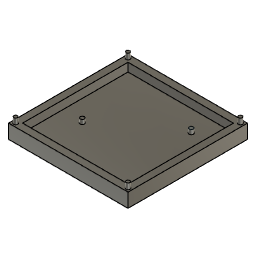
Untitled v0 (Autodesk Fusion 360 design; units mm, degrees)
Autodesk Fusion 360 part; units mm, degrees
note: some values were not read from the file. Set by a fixed rule: which sketch regions a step uses.
sketch "Sketch1" plane through (0, 0, 0) normal (0, 0, 1) x (1, 0, 0)
  line L0 (0, 0) -> (0, 75)
  line L1 (0, 75) -> (75, 75)
  line L2 (75, 75) -> (75, 0)
  line L3 (75, 0) -> (0, 0)
  line L4 (-5, -5) -> (-5, 80)
  line L5 (-5, 80) -> (80, 80)
  line L6 (80, 80) -> (80, -5)
  line L7 (80, -5) -> (-5, -5)
  dimension "d1" = 75
  dimension "d2" = 75
  dimension "d3" = 75
  dimension "d4" = 75
  dimension "d5" = 85
  dimension "d6" = 85
  dimension "d7" = 85
  dimension "d8" = 85
  constraint coincident L0.start L3.end
  constraint vertical L0
  constraint perpendicular L0 L1
  constraint perpendicular L1 L2
  constraint perpendicular L0 L3
  constraint parallel L0 L4
  constraint perpendicular L4 L5
  constraint perpendicular L5 L6
  constraint perpendicular L4 L7
  measures "d1" distance of L0.start L0.end
  measures "d2" distance of L0.end L1.end
  measures "d3" distance of L1.end L2.end
  measures "d4" distance of L2.end L0.start
  measures "d5" distance of L4.start L4.end
  measures "d6" distance of L4.end L5.end
  measures "d7" distance of L5.end L6.end
  measures "d8" distance of L6.end L4.start
extrude "Extrude1" add sketch "Sketch1" along normal blind 10
sketch "Sketch2" plane through (0, 0, 0) normal (0, 1, 0) x (1, 0, 0)
sketch "Sketch3" plane through (0, 0, 0) normal (0, 0, 1) x (1, 0, 0)
  line L0 (0, 0) -> (75, 0)
  line L1 (75, 0) -> (75, 75)
  line L2 (75, 75) -> (0, 75)
  line L3 (0, 75) -> (0, 0)
  constraint horizontal L0
  constraint vertical L1
  constraint horizontal L2
  constraint vertical L3
  constraint coincident L0.start L3.end
extrude "Extrude2" add sketch "Sketch3" along normal blind 4
sketch "Sketch4" plane through (0, 0, 4) normal (0, 0, 1) x (-1, 0, 0)
  line L0 (0, -75) -> (0, 0)
  line L1 (0, 0) -> (-75, 0)
  line L2 (-75, 0) -> (-75, -75)
  line L3 (-75, -75) -> (0, -75)
  line L4 (0, 0) -> (-75, -75)
  line L5 (-75, 0) -> (0, -75)
  line L6 (-37.5, -37.5) -> (-37.5, -65)
  line L7 (-37.5, -37.5) -> (-65, -37.5)
  line L8 (-65, -37.5) -> (-65, -10)
  line L9 (-37.5, -65) -> (-10, -65)
  line L10 (-10, -65) -> (-65, -65)
  line L11 (-65, -65) -> (-65, -10)
  line L12 (-65, -10) -> (-10, -10)
  line L13 (-10, -10) -> (-10, -65)
  line L14 (-65, -65) -> (-60, -65)
  line L15 (-60, -65) -> (-60, -60)
  circle A0 centre (-60, -60) radius 1.625
  line L16 (-10, -10) -> (-10, -27.5)
  line L17 (-10, -27.5) -> (-15, -27.5)
  circle A1 centre (-15, -27.5) radius 1.625
  dimension "d13" = 27.5
  dimension "d14" = 27.5
  dimension "d15" = 27.5
  dimension "d16" = 27.5
  dimension "d17" = 5
  dimension "d18" = 5
  dimension "d19" = 3.25
  dimension "d20" = 17.5
  dimension "d21" = 5
  dimension "d22" = 3.25
  constraint coincident L0.end L1.start
  constraint coincident L2.end L3.start
  constraint coincident L1.end L2.start
  constraint coincident L0.start L3.end
  constraint midpoint L4 L6.start
  constraint vertical L6
  constraint perpendicular L6 L7
  constraint perpendicular L7 L8
  constraint perpendicular L6 L9
  constraint horizontal L10
  constraint vertical L11
  constraint horizontal L12
  constraint vertical L13
  constraint perpendicular L11 L14
  constraint perpendicular L10 L15
  constraint coincident L15.end A0.centre
  constraint perpendicular L12 L16
  constraint perpendicular L13 L17
  constraint coincident L17.end A1.centre
  measures "d13" distance of L6.start L6.end
  measures "d14" distance of L6.start L7.end
  measures "d15" distance of L7.end L8.end
  measures "d16" distance of L6.end L9.end
  measures "d17" distance of L10.end L14.end
  measures "d18" distance of L14.end L15.end
  measures "d19" diameter of A0
  measures "d20" distance of L12.end L16.end
  measures "d21" distance of L16.end L17.end
  measures "d22" diameter of A1
extrude "Extrude3" add sketch "Sketch4" along normal blind 3 draft -4 contours L4 A0 | L4 L15 A0 | L4 L15 A0 | A1
sketch "Sketch5" plane through (0, 0, 10) normal (0, 0, 1) x (-1, 0, 0)
  line L0 (-75, -75) -> (-75, 0)
  line L1 (-75, 0) -> (0, 0)
  line L2 (0, 0) -> (0, -75)
  line L3 (0, -75) -> (-75, -75)
  line L4 (-80, 5) -> (-80, -80)
  line L5 (-80, -80) -> (5, -80)
  line L6 (5, -80) -> (5, 5)
  line L7 (5, 5) -> (-80, 5)
  line L8 (5, 5) -> (0, 0)
  line L9 (5, 0) -> (0, 5)
  circle A0 centre (2.5, 2.5) radius 1.5
  line L10 (-75, -75) -> (-80, -80)
  line L11 (-80, -75) -> (-75, -80)
  circle A1 centre (-77.5, -77.5) radius 1.5
  line L12 (0, -75) -> (5, -80)
  line L13 (5, -75) -> (0, -80)
  circle A2 centre (2.5, -77.5) radius 1.5
  line L14 (-80, 5) -> (-75, 0)
  line L15 (-75, 5) -> (-80, 0)
  circle A3 centre (-77.5, 2.5) radius 1.5
  dimension "d25" = 3
  dimension "d26" = 3
  dimension "d27" = 3
  dimension "d28" = 3
  constraint coincident L6.end L7.start
  constraint coincident L1.end L2.start
  constraint coincident L6 L9.start
  constraint coincident L7 L9.end
  constraint perpendicular L8 L9
  constraint midpoint L8 A0.centre
  constraint coincident L0.start L3.end
  constraint coincident L4.end L5.start
  constraint coincident L4 L11.start
  constraint coincident L5 L11.end
  constraint perpendicular L10 L11
  constraint midpoint L11 A1.centre
  constraint coincident L2.end L3.start
  constraint coincident L5.end L6.start
  constraint coincident L6 L13.start
  constraint coincident L5 L13.end
  constraint perpendicular L12 L13
  constraint midpoint L12 A2.centre
  constraint coincident L4.start L7.end
  constraint coincident L0.end L1.start
  constraint coincident L7 L15.start
  constraint coincident L4 L15.end
  constraint perpendicular L14 L15
  constraint midpoint L14 A3.centre
  measures "d25" diameter of A0
  measures "d26" diameter of A1
  measures "d27" diameter of A2
  measures "d28" diameter of A3
extrude "Extrude4" add sketch "Sketch5" along normal blind 4 draft -3 contours L10 L11 A1 | L10 L11 A1 | L14 L15 A3 | L14 L15 A3 | L12 L13 A2 | L12 L13 A2 | L10 L11 A1 | L10 L11 A1 | L8 L9 A0 | L8 L9 A0 | L14 L15 A3 | L14 L15 A3 | L12 L13 A2 | L12 L13 A2 | L8 L9 A0 | L8 L9 A0
sketch "Sketch6" plane through (0, 0, 7) normal (0, 0, 1) x (-1, 0, 0)
  circle A0 centre (-60, -60) radius 1.4152
equation "d13 = ( 55 / 2 ) * 1 mm"
equation "d14 = ( 55 / 2 ) * 1 mm"
equation "d15 = ( 55 / 2 ) * 1 mm"
equation "d16 = ( 55 / 2 ) * 1 mm"
